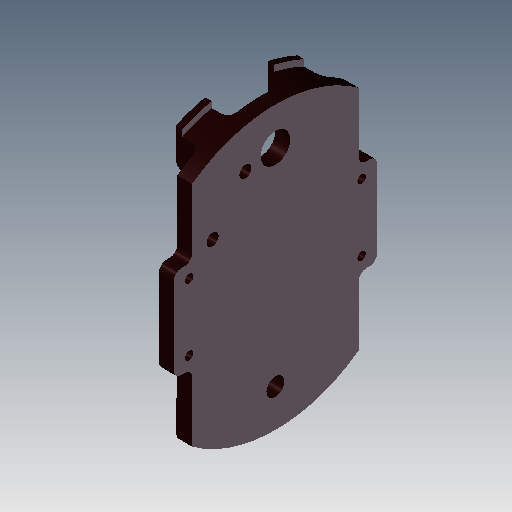
# Autodesk Inventor part: bottom_cap
Saved by Autodesk Inventor 2018 (Build 220112000, 112)
## iProperties
Created: 2018-12-05
Part Number: bottom_cap
Material: Generic
Document SubType Name: Modeling
Designer: Koki
Density: 1 g/cm^3
Appearance: Chestnut
Author: Koki
Autodesk Inventor part; units mm, degrees
ref_plane "YZ Plane" through (0, 0, 0) normal (1, 0, 0) x (0, 1, 0)
ref_plane "XZ Plane" through (0, 0, 0) normal (0, 1, 0) x (-1, 0, 0)
ref_plane "XY Plane" through (0, 0, 0) normal (0, 0, 1) x (1, 0, 0)
sketch "Sketch1" plane through (0, 0, 0) normal (1, 0, 0) x (0, 1, 0)
  line L0 (12.5, 27.5) -> (-12.5, 27.5)
  line L1 (-12.5, 27.5) -> (-12.5, -27.5)
  line L2 (-12.5, -27.5) -> (12.5, -27.5)
  line L3 (12.5, -27.5) -> (12.5, 27.5)
  point P0 (0, 0)
  dimension "d0" = 55
  dimension "d1" = 25
  dimension "d2" = 27.5
  dimension "d3" = 12.5
  constraints: 8 end point, 2 parallel, 1 horizontal, 1 perpendicular
  measures "d0" distance of L2.end L0.start
  measures "d1" distance of L0.start L0.end
  measures "d2" distance from line of point (0, 0) L0
  measures "d3" distance from line of point (0, 0) L3
extrude "Extrusion1" add sketch "Sketch1" along normal blind 4
sketch "Sketch2" plane through (4, 0, 0) normal (1, 0, 0) x (0, 0, -1)
  circle A0 centre (-23.3, 9) radius 1.15
  circle A1 centre (-23.3, -9) radius 1.15
  line L0 (-27.5, 12.5) -> (-27.5, -12.5) projected
  point P0 (0, 0)
  dimension "d6" = 2.3
  dimension "d7" = 2.3
  dimension "d8" = 18
  dimension "d9" = 9
  dimension "d10" = 4.2
  dimension "d11" = 4.2
  constraints: 2 centre point
  measures "d6" diameter of A0
  measures "d7" diameter of A1
  measures "d8" distance of A1.centre A0.centre
  measures "d9" vertical distance of point (0, 0) A0.centre
  measures "d10" distance from line of L0 A0.centre
  measures "d11" distance from line of L0 A1.centre
extrude "Extrusion2" cut sketch "Sketch2" against normal through all
mirror "Mirror1" about plane through (0, 0, 0) normal (0, 0, 1) of "Extrusion2"
sketch "Sketch3" plane through (4, 0, 0) normal (1, 0, 0) x (0, 0, -1)
  circle A0 centre (0, 0) radius 38.1
  line L0 (-22.5, 30.7467) -> (-22.5, -30.7467)
  line L1 (22.5, 30.7467) -> (22.5, -30.7467)
  line L2 (22.5, 12.5) -> (-22.5, 12.5)
  line L3 (27.5, 12.5) -> (-27.5, 12.5) projected
  dimension "d14" = 76.2
  dimension "d15" = 45
  dimension "d16" = 22.5
  constraints: 6 end point, 4 point on circle, 3 point on line, 2 vertical, 1 centre point, 1 coincident, 1 perpendicular
  measures "d14" diameter of A0
  measures "d15" distance between parallel lines of L1 L0
  measures "d16" distance from line of point (0, 0) L0
extrude "Extrusion4" add sketch "Sketch3" against normal blind 4 contours L1 L2 L0 A0 picked at (0, 21.0333)
mirror "Mirror2" about plane through (0, 0, 0) normal (0, 1, 0) of "Extrusion4"
sketch "Sketch6" plane through (0, 0, 0) normal (-1, 0, 0) x (0, 0, 1)
  arc A0 (-22.5, -30.7467) -> (22.5, -30.7467) centre (0, 0) ccw projected
  line L0 (16.5, -34.3418) -> (16.5, -26.3418)
  line L1 (8.5, -37.1397) -> (8.5, -26.3418)
  line L2 (16.5, -26.3418) -> (8.5, -26.3418)
  line L3 (22.5, -12.5) -> (22.5, -30.7467) projected
  dimension "d29" = 8
  dimension "d30" = 6
  dimension "d31" = 8
  constraints: 6 end point, 2 point on circle, 2 vertical, 1 perpendicular
  measures "d29" distance between parallel lines of L1 L0
  measures "d30" distance between parallel lines of L3 L0
  measures "d31" distance of L0.start L0.end
extrude "Extrusion6" add sketch "Sketch6" along normal blind 6.5
sketch "Sketch7" plane through (-6.5, 0, 0) normal (-1, 0, 0) x (0, 0, 1)
  arc A0 (8.5, -37.1397) -> (16.5, -34.3418) centre (0, 0) ccw projected
  circle A1 centre (0, 0) radius 39.6875
  line L0 (16.5, -36.095) -> (16.5, -34.3418)
  line L1 (8.5, -38.7666) -> (8.5, -37.1397)
  dimension "d34" = 79.375
  constraints: 4 end point, 2 point on circle, 2 vertical, 1 centre point, 1 coincident
  measures "d34" diameter of A1
extrude "Extrusion7" add sketch "Sketch7" against normal blind 1.75 contours A0 L0 A1 L1 picked at (15.635, -35.3029)
mirror "Mirror3" about plane through (0, 0, 0) normal (0, 0, 1) of "Extrusion6", "Extrusion7"
mirror "Mirror4" about plane through (0, 0, 0) normal (0, 1, 0) of "Extrusion6", "Extrusion7", "Mirror3"
fillet "Fillet1" radius 2 4 edges at (2, -12.5, 22.5) (2, 12.5, 22.5) (2, 12.5, -22.5) (2, -12.5, -22.5)
fillet "Fillet2" radius 2 4 edges at (2, 12.5, 27.5) (2, -12.5, 27.5) (2, -12.5, -27.5) (2, 12.5, -27.5)
fillet "Fillet3" radius 2 12 edges at (0, -30.3418, 16.5) (0, -31.7408, -8.5) (0, -31.7408, 8.5) (0, -26.3418, 12.5) (0, -26.3418, -12.5) (0, -30.3418, -16.5) (0, 30.3418, -16.5) (0, 31.7408, -8.5) (0, 26.3418, -12.5) (0, 31.7408, 8.5) (0, 26.3418, 12.5) (0, 30.3418, 16.5)
fillet "Fillet4" radius 2 4 edges at (-6.5, -26.3418, 12.5) (-6.5, -26.3418, -12.5) (-6.5, 26.3418, -12.5) (-6.5, 26.3418, 12.5)
sketch "Sketch8" plane through (4, 0, 0) normal (1, 0, 0) x (0, 0, -1)
  circle A0 centre (-17, 15) radius 1.651
  circle A1 centre (-8.11, 26.43) radius 1.651
  point P0 (0, 0)
  dimension "d42" = 3.302
  dimension "d43" = 15
  dimension "d44" = 17
  dimension "d45" = 3.302
  dimension "d46" = 8.89
  dimension "d47" = 11.43
  constraints: 2 centre point
  measures "d42" diameter of A0
  measures "d43" vertical distance of point (0, 0) A0.centre
  measures "d44" horizontal distance of point (0, 0) A0.centre
  measures "d45" diameter of A1
  measures "d46" horizontal distance of A1.centre A0.centre
  measures "d47" vertical distance of A0.centre A1.centre
extrude "Extrusion8" cut sketch "Sketch8" against normal blind 10
sketch "Sketch9" plane through (4, 0, 0) normal (1, 0, 0) x (0, 0, -1)
  line L0 (0, 0) -> (11.5705, 0)
  circle A0 centre (0, -27.94) radius 2.425
  circle A1 centre (0, 27.94) radius 4
  dimension "d50" = 4.85
  dimension "d51" = 27.94
  dimension "d62" = 8
  constraints: 2 centre point, 2 end point, 1 horizontal, 1 symmetric about line
  measures "d50" diameter of A0
  measures "d51" distance from line of A0.centre L0
  measures "d62" diameter of A1
extrude "Extrusion9" cut sketch "Sketch9" against normal blind 10
sketch "Sketch10" plane through (0, 0, 0) normal (-1, 0, 0) x (0, 0, 1)
  circle A0 centre (8.11, 26.43) radius 1.651 projected
  line L0 (4.3572, 26.43) -> (6.2336, 29.68)
  line L1 (6.2336, 29.68) -> (9.9864, 29.68)
  line L2 (9.9864, 29.68) -> (11.8628, 26.43)
  line L3 (11.8628, 26.43) -> (9.9864, 23.18)
  line L4 (9.9864, 23.18) -> (6.2336, 23.18)
  line L5 (6.2336, 23.18) -> (4.3572, 26.43)
  point P0 (0, 0)
  dimension "d54" = 6.5
  constraints: 12 end point, 1 coincident, 1 horizontal, 13 other
  measures "d54" distance between parallel lines of L3 L0
extrude "Extrusion10" cut sketch "Sketch10" along normal blind 10 contours A0 | L0 L1 L2 L3 L4 L5
equation "\"d2\" = 0.5 * d0"
equation "\"d3\" = 0.5 * d1"
equation "\"d9\" = 0.5 * d8"
equation "\"d11\" = d10"
equation "\"d16\" = 0.5 * d15"
equation "\"d45\" = d42"
body "Solid1"
